Autodesk Fusion 360 part; units mm, degrees
note: some values were not read from the file. Chosen so that the rebuilt part matches the saved one: a direction; which face or edge a step refers to; a side. Set by a fixed rule: which sketch regions a step uses.
(part 2 of 2)
extrude "Extrusion31" cut sketch "Skizze28" against normal blind 1.5 contours L3 A2 A3 | L3 A2 A3 | L3 A3 picked at (-0.3969, 21.4267) bodies 2
sketch "Skizze29" plane through (0, 1.5, 0) normal (0, 1, 0) x (-1, 0, 0)
  line L0 (0.5, -16) -> (0.5, -41)
  line L1 (0.5, -41) -> (35.5, -41)
  line L2 (35.5, -41) -> (35.5, -11)
  line L3 (61, -16) -> (61, -41)
  line L4 (61, -41) -> (67.5, -41)
  line L5 (67.5, -41) -> (67.5, 41)
  line L6 (67.5, 41) -> (38.5, 41)
  line L7 (-67.5, 41) -> (-67.5, -41)
  line L8 (-67.5, -41) -> (-25, -41)
  line L9 (-25, -41) -> (-25, -16)
  line L10 (-25, -16) -> (0.5, -16)
  line L11 (38.5, 33) -> (32.5, 33)
  line L12 (32.5, 33) -> (32.5, 41)
  line L13 (38.5, 41) -> (38.5, 33)
  line L14 (-38.5, -5) -> (-32.5, -5)
  line L15 (-32.5, -5) -> (-32.5, -11)
  line L16 (-38.5, -11) -> (-38.5, -5)
  line L17 (-67.5, -11) -> (-57.5, -11)
  line L18 (-57.5, -11) -> (-57.5, 19)
  line L19 (-57.5, 19) -> (-67.5, 19)
  line L20 (-67.5, 19) -> (-67.5, -11)
  line L21 (-67.5, -11.5) -> (-56.5, -11.5)
  line L22 (-56.5, -11.5) -> (-56.5, -9.5)
  line L23 (-56.5, -9.5) -> (-54.5, -9.5)
  line L24 (-54.5, -9.5) -> (-54.5, -13.5)
  line L25 (-54.5, -13.5) -> (-67.5, -13.5)
  line L26 (-67.5, 19.5) -> (-57, 19.5)
  line L27 (-57, 19.5) -> (-57, 17.5)
  line L28 (-57, 17.5) -> (-55, 17.5)
  line L29 (-55, 17.5) -> (-55, 21.5)
  line L30 (-55, 21.5) -> (-67.5, 21.5)
  line L31 (-38.5, 35) -> (-38.5, 41)
  line L32 (-34.5, 41) -> (-34.5, 35)
  line L33 (-34.5, 35) -> (-38.5, 35)
  line L34 (38.5, -7) -> (38.5, -16)
  line L35 (34.5, -11) -> (34.5, -7)
  line L36 (34.5, -7) -> (38.5, -7)
  line L37 (38.5, -16) -> (61, -16)
  line L38 (32.5, 41) -> (-34.5, 41)
  line L39 (-38.5, 41) -> (-67.5, 41)
  line L40 (35.5, -11) -> (34.5, -11)
  line L41 (-32.5, -11) -> (-38.5, -11)
  dimension "d194" = 1
  dimension "d195" = 0.5
  dimension "d196" = 2
  dimension "d197" = 2
  dimension "d198" = 1.5
  dimension "d199" = 0.5
  dimension "d200" = 0.5
  dimension "d201" = 2
  dimension "d202" = 2
  dimension "d203" = 1.5
  constraint coincident L7 L21.start
  constraint perpendicular L7 L21
  constraint perpendicular L21 L22
  constraint perpendicular L7 L23
  constraint perpendicular L23 L24
  constraint coincident L7 L25.end
  constraint perpendicular L7 L25
  constraint coincident L7 L26.start
  constraint perpendicular L7 L26
  constraint perpendicular L26 L27
  constraint perpendicular L7 L28
  constraint perpendicular L26 L29
  constraint coincident L7 L30.end
  constraint perpendicular L7 L30
  measures "d194" distance of L18 L22
  measures "d195" distance of L17 L21
  measures "d196" distance of L21 L25
  measures "d197" distance of L22 L24
  measures "d198" distance of L17 L23
  measures "d199" distance of L19 L26
  measures "d200" distance of L18 L27
  measures "d201" distance of L26 L30
  measures "d202" distance of L27 L29
  measures "d203" distance of L19 L28
extrude "Extrusion32" add sketch "Skizze29" along normal up to surface (12.5 mm away) contours L7 L21 L22 L23 L24 L25 | L7 L26 L27 L28 L29 L30 bodies 1
sketch "Skizze30" plane through (0, 0, 42.5) normal (0, 0, 1) x (1, 0, 0)
  line L0 (29.5, 41.5) -> (29.5, 34.5)
  line L1 (29.5, 34.5) -> (16.5, 34.5)
  line L2 (16.5, 34.5) -> (16.5, 41.5)
  line L3 (16.5, 41.5) -> (-48, 41.5)
  line L4 (-48, 41.5) -> (-69, 20.5)
  line L5 (-69, 20.5) -> (-69, 14)
  line L6 (-69, 14) -> (69, 14)
  line L7 (69, 14) -> (69, 32.5)
  line L8 (69, 32.5) -> (60, 41.5)
  line L9 (60, 41.5) -> (29.5, 41.5)
  line L10 (-29.7713, 17.8604) -> (-38.3749, 30.1476)
  arc A0 (-38.3749, 30.1476) -> (-40.8324, 28.4269) centre (-39.6036, 29.2873) ccw
  line L11 (-40.8324, 28.4269) -> (-32.2287, 16.1396)
  arc A1 (-32.2287, 16.1396) -> (-29.7713, 17.8604) centre (-31, 17) ccw
  line L12 (-31, 17) -> (-39.6036, 29.2873) construction
  line L13 (-28.8324, 28.4269) -> (-20.2287, 16.1396)
  arc A2 (-26.3749, 30.1476) -> (-28.8324, 28.4269) centre (-27.6036, 29.2873) ccw
  line L14 (-17.7713, 17.8604) -> (-26.3749, 30.1476)
  arc A3 (-20.2287, 16.1396) -> (-17.7713, 17.8604) centre (-19, 17) ccw
  line L15 (-16.8324, 28.4269) -> (-8.2287, 16.1396)
  arc A4 (-14.3749, 30.1476) -> (-16.8324, 28.4269) centre (-15.6036, 29.2873) ccw
  line L16 (-5.7713, 17.8604) -> (-14.3749, 30.1476)
  arc A5 (-8.2287, 16.1396) -> (-5.7713, 17.8604) centre (-7, 17) ccw
  line L17 (-4.8324, 28.4269) -> (3.7713, 16.1396)
  line L18 (6.2287, 17.8604) -> (-2.3749, 30.1476)
  arc A6 (-2.3749, 30.1476) -> (-4.8324, 28.4269) centre (-3.6036, 29.2873) ccw
  arc A7 (3.7713, 16.1396) -> (6.2287, 17.8604) centre (5, 17) ccw
  line L19 (54.2287, 17.8604) -> (45.6251, 30.1476)
  line L20 (43.1676, 28.4269) -> (51.7713, 16.1396)
  arc A8 (51.7713, 16.1396) -> (54.2287, 17.8604) centre (53, 17) ccw
  arc A9 (45.6251, 30.1476) -> (43.1676, 28.4269) centre (44.3964, 29.2873) ccw
  line L21 (42.2287, 17.8604) -> (33.6251, 30.1476)
  line L22 (31.1676, 28.4269) -> (39.7713, 16.1396)
  arc A10 (33.6251, 30.1476) -> (31.1676, 28.4269) centre (32.3964, 29.2873) ccw
  arc A11 (39.7713, 16.1396) -> (42.2287, 17.8604) centre (41, 17) ccw
  line L23 (30.2287, 17.8604) -> (21.6251, 30.1476)
  arc A12 (27.7713, 16.1396) -> (30.2287, 17.8604) centre (29, 17) ccw
  line L24 (19.1676, 28.4269) -> (27.7713, 16.1396)
  arc A13 (21.6251, 30.1476) -> (19.1676, 28.4269) centre (20.3964, 29.2873) ccw
  line L25 (18.2287, 17.8604) -> (9.6251, 30.1476)
  line L26 (7.1676, 28.4269) -> (15.7713, 16.1396)
  arc A14 (15.7713, 16.1396) -> (18.2287, 17.8604) centre (17, 17) ccw
  arc A15 (9.6251, 30.1476) -> (7.1676, 28.4269) centre (8.3964, 29.2873) ccw
  line L27 (-69, 14) -> (69, 14)
  line L28 (69, 14) -> (69, 17)
  line L29 (69, 17) -> (-69, 17)
  line L30 (-69, 17) -> (-69, 14)
  dimension "d206" = 15
  dimension "d207" = 3
  dimension "d208" = 15
  dimension "d209" = 3
  dimension "d210" = 15
  dimension "d211" = 3
  dimension "d212" = 15
  dimension "d213" = 3
  dimension "d214" = 15
  dimension "d215" = 3
  dimension "d216" = 15
  dimension "d217" = 3
  dimension "d218" = 15
  dimension "d219" = 3
  dimension "d220" = 15
  dimension "d221" = 3
  dimension "d222" = 3
  dimension "d224" = 12
  dimension "d225" = 12
  dimension "d226" = 12
  dimension "d227" = 12
  dimension "d228" = 12
  dimension "d229" = 12
  dimension "d230" = 12
  dimension "d231" = 38
  dimension "d234" = 55
  constraint tangent L10 A0
  constraint tangent A0 L11
  constraint parallel L10 L11
  constraint tangent L11 A1
  constraint tangent L10 A1
  constraint tangent A2 L14
  constraint tangent L13 A2
  constraint parallel L13 L14
  constraint tangent L13 A3
  constraint tangent L14 A3
  constraint tangent A4 L16
  constraint tangent L15 A4
  constraint parallel L15 L16
  constraint tangent L15 A5
  constraint tangent L16 A5
  constraint tangent L18 A6
  constraint tangent L17 A6
  constraint parallel L17 L18
  constraint tangent L17 A7
  constraint tangent L18 A7
  constraint tangent L25 A15
  constraint tangent L26 A15
  constraint parallel L25 L26
  constraint tangent L26 A14
  constraint tangent L25 A14
  constraint tangent L23 A13
  constraint tangent L24 A13
  constraint parallel L23 L24
  constraint tangent A12 L24
  constraint tangent L23 A12
  constraint tangent L21 A10
  constraint tangent L22 A10
  constraint parallel L21 L22
  constraint tangent L22 A11
  constraint tangent L21 A11
  constraint tangent L19 A9
  constraint tangent L20 A9
  constraint parallel L19 L20
  constraint tangent L20 A8
  constraint tangent L19 A8
  constraint horizontal L27
  constraint vertical L28
  constraint horizontal L29
  constraint vertical L30
  constraint coincident L7 L28.end
  constraint coincident L5.end L6.start
  constraint coincident A1.centre L29
  constraint coincident A3.centre L29
  constraint coincident A5.centre L29
  constraint coincident A7.centre L29
  constraint coincident A14.centre L29
  constraint coincident A12.centre L29
  constraint coincident A11.centre L29
  constraint coincident A8.centre L29
  constraint parallel L10 L13
  constraint parallel L14 L15
  constraint parallel L16 L17
  constraint parallel L18 L26
  constraint parallel L24 L25
  constraint parallel L22 L23
  constraint parallel L20 L21
  measures "d206" distance of A1.centre A0.centre
  measures "d207" diameter of A0
  measures "d208" distance of A2.centre A3.centre
  measures "d209" diameter of A2
  measures "d210" distance of A4.centre A5.centre
  measures "d211" diameter of A4
  measures "d212" distance of A6.centre A7.centre
  measures "d213" diameter of A6
  measures "d214" distance of A15.centre A14.centre
  measures "d215" diameter of A15
  measures "d216" distance of A13.centre A12.centre
  measures "d217" diameter of A13
  measures "d218" distance of A10.centre A11.centre
  measures "d219" diameter of A10
  measures "d220" distance of A9.centre A8.centre
  measures "d221" diameter of A9
  measures "d222" distance of L27 L29
  measures "d224" distance of A1.centre A3.centre
  measures "d225" distance of A3.centre A5.centre
  measures "d226" distance of A5.centre A7.centre
  measures "d227" distance of A7.centre A14.centre
  measures "d228" distance of A14.centre A12.centre
  measures "d229" distance of A12.centre A11.centre
  measures "d230" distance of A11.centre A8.centre
  measures "d231" distance of A1.centre L29.end
  measures "d234" angle of L11 L29
extrude "Extrusion33" cut sketch "Skizze30" against normal blind 1.5 contours L19 L20 A8 A9 L29 | L20 A8 L29 | L21 L22 A10 A11 L29 | L22 A11 L29 | L11 A1 L29 | L10 A0 L11 A1 L29 | L23 A12 L24 A13 L29 | A12 L24 L29 | L13 A3 L29 | L13 A2 L14 A3 L29 | L25 L26 A14 A15 L29 | L26 A14 L29 | L15 A5 L29 | L15 A4 L16 A5 L29 | L17 L18 A6 A7 L29 | L17 A7 L29 bodies 2
sketch "Skizze34" plane through (0, 0, 42.5) normal (0, 0, 1) x (1, 0, 0)
  line L0 (27.7713, 16.1396) -> (19.1676, 28.4269)
  arc A0 (21.6251, 30.1476) -> (19.1676, 28.4269) centre (20.3964, 29.2873) ccw
  line L1 (21.6251, 30.1476) -> (30.2287, 17.8604)
  arc A1 (27.7713, 16.1396) -> (30.2287, 17.8604) centre (29, 17) ccw
  line L2 (-26.3749, 30.1476) -> (-17.7713, 17.8604)
  arc A2 (-20.2287, 16.1396) -> (-17.7713, 17.8604) centre (-19, 17) ccw
  line L3 (-20.2287, 16.1396) -> (-28.8324, 28.4269)
  arc A3 (-26.3749, 30.1476) -> (-28.8324, 28.4269) centre (-27.6036, 29.2873) ccw
  line L4 (-14.3749, 30.1476) -> (-5.7713, 17.8604)
  arc A4 (-8.2287, 16.1396) -> (-5.7713, 17.8604) centre (-7, 17) ccw
  line L5 (-8.2287, 16.1396) -> (-16.8324, 28.4269)
  arc A5 (-14.3749, 30.1476) -> (-16.8324, 28.4269) centre (-15.6036, 29.2873) ccw
  line L6 (33.6251, 30.1476) -> (42.2287, 17.8604)
  arc A6 (39.7713, 16.1396) -> (42.2287, 17.8604) centre (41, 17) ccw
  line L7 (39.7713, 16.1396) -> (31.1676, 28.4269)
  arc A7 (33.6251, 30.1476) -> (31.1676, 28.4269) centre (32.3964, 29.2873) ccw
  line L8 (15.7713, 16.1396) -> (7.1676, 28.4269)
  arc A8 (9.6251, 30.1476) -> (7.1676, 28.4269) centre (8.3964, 29.2873) ccw
  line L9 (9.6251, 30.1476) -> (18.2287, 17.8604)
  arc A9 (15.7713, 16.1396) -> (18.2287, 17.8604) centre (17, 17) ccw
  line L10 (-38.3749, 30.1476) -> (-29.7713, 17.8604)
  arc A10 (-32.2287, 16.1396) -> (-29.7713, 17.8604) centre (-31, 17) ccw
  line L11 (-32.2287, 16.1396) -> (-40.8324, 28.4269)
  arc A11 (-38.3749, 30.1476) -> (-40.8324, 28.4269) centre (-39.6036, 29.2873) ccw
  line L12 (-2.3749, 30.1476) -> (6.2287, 17.8604)
  arc A12 (3.7713, 16.1396) -> (6.2287, 17.8604) centre (5, 17) ccw
  line L13 (3.7713, 16.1396) -> (-4.8324, 28.4269)
  arc A13 (-2.3749, 30.1476) -> (-4.8324, 28.4269) centre (-3.6036, 29.2873) ccw
  line L14 (51.7713, 16.1396) -> (43.1676, 28.4269)
  arc A14 (45.6251, 30.1476) -> (43.1676, 28.4269) centre (44.3964, 29.2873) ccw
  line L15 (45.6251, 30.1476) -> (54.2287, 17.8604)
  arc A15 (51.7713, 16.1396) -> (54.2287, 17.8604) centre (53, 17) ccw
  line L16 (29.5, 41.5) -> (29.5, 34.5)
  line L17 (29.5, 34.5) -> (16.5, 34.5)
  line L18 (16.5, 34.5) -> (16.5, 41.5)
  line L19 (16.5, 41.5) -> (-48, 41.5)
  line L20 (-48, 41.5) -> (-69, 20.5)
  line L21 (-69, 20.5) -> (-69, 14)
  line L22 (-69, 14) -> (69, 14)
  line L23 (69, 14) -> (69, 32.5)
  line L24 (69, 32.5) -> (60, 41.5)
  line L25 (60, 41.5) -> (29.5, 41.5)
  line L26 (48, 41.5) -> (69, 20.5)
  dimension "d239" = 45
  dimension "d240" = 21
  constraint coincident L25 L26.start
  constraint coincident L23 L26.end
  measures "d239" angle of L25 L26
  measures "d240" distance of L23 L26.start
extrude "Extrusion36" cut sketch "Skizze34" against normal up to surface (22.5 mm away) contours L23 L24 L25 L26 bodies 2
sketch "Skizze35" plane through (0, 0, -42.5) normal (0, 0, -1) x (-1, 0, 0)
  line L0 (11.7592, 31.0652) -> (2.0084, 17.1396)
  arc A0 (-0.449, 18.8604) -> (2.0084, 17.1396) centre (0.7797, 18) ccw
  line L1 (-0.449, 18.8604) -> (9.3018, 32.7859)
  arc A1 (11.7592, 31.0652) -> (9.3018, 32.7859) centre (10.5305, 31.9256) ccw
  line L2 (-24.4169, 31.0652) -> (-34.1677, 17.1396)
  arc A2 (-36.6251, 18.8604) -> (-34.1677, 17.1396) centre (-35.3964, 18) ccw
  line L3 (-36.6251, 18.8604) -> (-26.8743, 32.7859)
  arc A3 (-24.4169, 31.0652) -> (-26.8743, 32.7859) centre (-25.6456, 31.9256) ccw
  arc A4 (23.4355, 31.0652) -> (20.978, 32.7859) centre (22.2067, 31.9256) ccw
  line L4 (23.4355, 31.0652) -> (13.6847, 17.1396)
  arc A5 (11.2272, 18.8604) -> (13.6847, 17.1396) centre (12.4559, 18) ccw
  line L5 (11.2272, 18.8604) -> (20.978, 32.7859)
  line L6 (-12.4933, 18.8604) -> (-2.7425, 32.7859)
  arc A6 (-0.285, 31.0652) -> (-2.7425, 32.7859) centre (-1.5137, 31.9256) ccw
  line L7 (-0.285, 31.0652) -> (-10.0358, 17.1396)
  arc A7 (-12.4933, 18.8604) -> (-10.0358, 17.1396) centre (-11.2645, 18) ccw
  line L8 (-12.202, 31.0652) -> (-21.9528, 17.1396)
  arc A8 (-24.4103, 18.8604) -> (-21.9528, 17.1396) centre (-23.1816, 18) ccw
  line L9 (-24.4103, 18.8604) -> (-14.6595, 32.7859)
  arc A9 (-12.202, 31.0652) -> (-14.6595, 32.7859) centre (-13.4308, 31.9256) ccw
  arc A10 (35.8961, 31.0652) -> (33.4386, 32.7859) centre (34.6674, 31.9256) ccw
  line L10 (35.8961, 31.0652) -> (26.1453, 17.1396)
  arc A11 (23.6878, 18.8604) -> (26.1453, 17.1396) centre (24.9166, 18) ccw
  line L11 (23.6878, 18.8604) -> (33.4386, 32.7859)
  line L12 (-69, 32.5) -> (-69, 14)
  line L13 (-69, 14) -> (69, 14)
  line L14 (69, 14) -> (69, 20.5)
  line L15 (69, 20.5) -> (48, 41.5)
  line L16 (48, 41.5) -> (-60, 41.5)
  line L17 (-60, 41.5) -> (-69, 32.5)
  line L18 (-48, 41.5) -> (-69, 20.5)
  dimension "d243" = 45
  dimension "d244" = 21
  constraint coincident L16 L18.start
  constraint coincident L12 L18.end
  measures "d243" angle of L16 L18
  measures "d244" distance of L12 L18.start
extrude "Extrusion37" cut sketch "Skizze35" against normal up to surface (30.5 mm away) contours L12 L16 L17 L18 bodies 2
sketch "Skizze36" plane through (44.75, 44.75, 0) normal (0.707107, 0.707107, 0) x (0, 0, -1)
  line L0 (-41, -6.7175) -> (-20, -6.7175)
  line L1 (-20, -6.7175) -> (-20, -4.5962)
  line L2 (-20, -4.5962) -> (-42.5, -4.5962)
  line L3 (-42.5, -4.5962) -> (-42.5, -34.2947)
  line L4 (-42.5, -34.2947) -> (-20, -34.2947)
  line L5 (-20, -34.2947) -> (-20, -32.1734)
  line L6 (-20, -32.1734) -> (-41, -32.1734)
  line L7 (-41, -32.1734) -> (-41, -6.7175)
  line L8 (-42.5, -4.5962) -> (-20, -4.5962)
  line L9 (-20, -4.5962) -> (-20, -34.2947)
  line L10 (-20, -34.2947) -> (-42.5, -34.2947)
  line L11 (-42.5, -34.2947) -> (-42.5, -4.5962)
  line L12 (12, -6.7175) -> (41, -6.7175)
  line L13 (41, -6.7175) -> (41, -32.1734)
  line L14 (41, -32.1734) -> (12, -32.1734)
  line L15 (12, -32.1734) -> (12, -34.2947)
  line L16 (12, -34.2947) -> (42.5, -34.2947)
  line L17 (42.5, -34.2947) -> (42.5, -4.5962)
  line L18 (42.5, -4.5962) -> (12, -4.5962)
  line L19 (12, -4.5962) -> (12, -6.7175)
  line L20 (12, -4.5962) -> (42.5, -4.5962)
  line L21 (42.5, -4.5962) -> (42.5, -34.2947)
  line L22 (42.5, -34.2947) -> (12, -34.2947)
  line L23 (12, -34.2947) -> (12, -4.5962)
  constraint horizontal L8
  constraint vertical L9
  constraint horizontal L10
  constraint vertical L11
  constraint coincident L4.end L5.start
  constraint coincident L2.end L3.start
  constraint horizontal L20
  constraint vertical L21
  constraint horizontal L22
  constraint vertical L23
  constraint coincident L16.end L17.start
  constraint coincident L18.end L19.start
extrude "Extrusion38" add sketch "Skizze36" against normal blind 1.5 bodies 2
sketch "Skizze37" plane through (0, 0, 20) normal (0, 0, 1) x (1, 0, 0)
  line L0 (49.5, 40) -> (59.3787, 40)
  line L1 (59.3787, 40) -> (67.5, 31.8787)
  line L2 (67.5, 31.8787) -> (67.5, 22)
  line L3 (67.5, 22) -> (69, 20.5)
  line L4 (69, 20.5) -> (69, 32.5)
  line L5 (69, 32.5) -> (60, 41.5)
  line L6 (60, 41.5) -> (48, 41.5)
  line L7 (48, 41.5) -> (49.5, 40)
  line L8 (49.5, 40) -> (67.5, 22)
extrude "Extrusion39" add sketch "Skizze37" along normal blind 1.5 bodies 2
sketch "Skizze38" plane through (0, 0, -12) normal (0, 0, -1) x (-1, 0, 0)
  line L0 (-59.3787, 40) -> (-49.5, 40)
  line L1 (-49.5, 40) -> (-48, 41.5)
  line L2 (-48, 41.5) -> (-60, 41.5)
  line L3 (-60, 41.5) -> (-69, 32.5)
  line L4 (-69, 32.5) -> (-69, 20.5)
  line L5 (-69, 20.5) -> (-67.5, 22)
  line L6 (-67.5, 22) -> (-67.5, 31.8787)
  line L7 (-67.5, 31.8787) -> (-59.3787, 40)
  line L8 (-67.5, 22) -> (-49.5, 40)
extrude "Extrusion40" add sketch "Skizze38" along normal blind 1.5 bodies 2
sketch "Skizze39" plane through (0, 1.5, 0) normal (0, 1, 0) x (-1, 0, 0)
  line L0 (-57, 19.5) -> (-67.5, 19.5)
  line L1 (-67.5, 19.5) -> (-67.5, -11.5)
  line L2 (-67.5, -11.5) -> (-56.5, -11.5)
  line L3 (-56.5, -11.5) -> (-56.5, -9.5)
  line L4 (-56.5, -9.5) -> (-54.5, -9.5)
  line L5 (-54.5, -9.5) -> (-54.5, -13.5)
  line L6 (-54.5, -13.5) -> (-67.5, -13.5)
  line L7 (-67.5, -13.5) -> (-67.5, -41)
  line L8 (-67.5, -41) -> (-25, -41)
  line L9 (-25, -41) -> (-25, -16)
  line L10 (-25, -16) -> (0.5, -16)
  line L11 (0.5, -16) -> (0.5, -41)
  line L12 (0.5, -41) -> (35.5, -41)
  line L13 (35.5, -41) -> (35.5, -11)
  line L14 (61, -16) -> (61, -41)
  line L15 (61, -41) -> (67.5, -41)
  line L16 (67.5, -41) -> (67.5, 41)
  line L17 (67.5, 41) -> (38.5, 41)
  line L18 (-67.5, 41) -> (-67.5, 21.5)
  line L19 (-67.5, 21.5) -> (-55, 21.5)
  line L20 (-55, 21.5) -> (-55, 17.5)
  line L21 (-55, 17.5) -> (-57, 17.5)
  line L22 (-57, 17.5) -> (-57, 19.5)
  line L23 (-38.5, -5) -> (-32.5, -5)
  line L24 (-32.5, -5) -> (-32.5, -11)
  line L25 (-38.5, -11) -> (-38.5, -5)
  line L26 (38.5, 33) -> (32.5, 33)
  line L27 (32.5, 33) -> (32.5, 41)
  line L28 (38.5, 41) -> (38.5, 33)
  line L29 (67.5, 41) -> (61.5, 41)
  line L30 (61.5, 41) -> (61.5, 36)
  line L31 (61.5, 36) -> (67.5, 36)
  line L32 (67.5, 36) -> (67.5, 41)
  circle A0 centre (64.5, 38.5) radius 1.6
  line L33 (0, 1.75) -> (0, 22.5)
  line L34 (-61.5, 41) -> (-61.5, 36)
  line L35 (-61.5, 36) -> (-67.5, 36)
  circle A1 centre (-64.5, 38.5) radius 1.6
  line L36 (-67.5, 41) -> (-61.5, 41)
  line L37 (-67.5, 36) -> (-67.5, 41)
  line L38 (-1.75, 0) -> (-22.5, 0)
  line L39 (61.5, -36) -> (67.5, -36)
  circle A2 centre (64.5, -38.5) radius 1.6
  line L40 (61.5, -41) -> (61.5, -36)
  line L41 (67.5, -41) -> (61.5, -41)
  line L42 (67.5, -36) -> (67.5, -41)
  line L43 (-61.5, -41) -> (-61.5, -36)
  line L44 (-61.5, -36) -> (-67.5, -36)
  line L45 (-67.5, -36) -> (-67.5, -41)
  line L46 (-67.5, -41) -> (-61.5, -41)
  circle A3 centre (-64.5, -38.5) radius 1.6
  line L47 (38.5, -7) -> (38.5, -16)
  line L48 (34.5, -11) -> (34.5, -7)
  line L49 (34.5, -7) -> (38.5, -7)
  line L50 (-38.5, 35) -> (-38.5, 41)
  line L51 (-34.5, 41) -> (-34.5, 35)
  line L52 (-34.5, 35) -> (-38.5, 35)
  line L53 (38.5, -16) -> (61, -16)
  line L54 (32.5, 41) -> (-34.5, 41)
  line L55 (-38.5, 41) -> (-67.5, 41)
  line L56 (35.5, -11) -> (34.5, -11)
  line L57 (-32.5, -11) -> (-38.5, -11)
  point P0 (-64.5, -38.5)
  point P1 (-64.5, -38.5)
  dimension "d253" = 6
  dimension "d254" = 5
  dimension "d255" = 3.2
  dimension "d256" = 3
  dimension "d257" = 2.5
  constraint horizontal L29
  constraint vertical L30
  constraint horizontal L31
  constraint vertical L32
  constraint coincident L16.end L17.start
  constraint symmetric L16.end L33 L18.start
  constraint symmetric L29.end L33 L34.start
  constraint symmetric L30.end L33 L34.end
  constraint symmetric L31.end L33 L35.end
  constraint symmetric A0 L33 A1
  constraint symmetric L16.end L38 L15.end
  constraint symmetric L29.end L38 L40.start
  constraint symmetric L30.end L38 L39.start
  constraint symmetric L31.end L38 L39.end
  constraint symmetric A0 L38 A2
  constraint symmetric L34.start L38 L43.start
  constraint symmetric L34.end L38 L43.end
  constraint symmetric L35.end L38 L44.end
  constraint symmetric A1.centre L38 P1
  constraint symmetric L18.start L38 L7.end
  constraint symmetric A1 L38 A3
  measures "d253" distance of L30.end L31.end
  measures "d254" distance of L29.end L30.end
  measures "d255" diameter of A0
  measures "d256" distance of L32 A0.centre
  measures "d257" distance of L31 A0.centre
extrude "Extrusion41" add sketch "Skizze39" along normal up to surface (11 mm away) contours L18 L34 L35 L36 L37 L55 | L7 L8 L43 L44 L45 L46 | L16 L17 L29 L30 L31 L32 | L15 L16 L39 L40 L41 L42 bodies 1
extrude "Extrusion58" cut 4 faces at (64.7139, 1.5, 38.603) (64.7139, 1.5, -38.397) (-64.1384, 1.5, 39.3056) (-64.1384, 1.5, -37.6944) along direction (0, 1, 0) up to surface end surface through (0, 0, 0) normal (0, -1, 0) offset 0 on bodies 1 bodies 1
sketch "Skizze54" plane through (0, 1.5, 0) normal (0, 1, 0) x (-1, 0, 0)
  line L0 (-61.5, 36) -> (-67.5, 36)
  line L1 (-67.5, 36) -> (-67.5, 21.5)
  line L2 (-67.5, 21.5) -> (-55, 21.5)
  line L3 (-55, 21.5) -> (-55, 17.5)
  line L4 (-55, 17.5) -> (-57, 17.5)
  line L5 (-57, 17.5) -> (-57, 19.5)
  line L6 (-57, 19.5) -> (-67.5, 19.5)
  line L7 (-67.5, 19.5) -> (-67.5, -11.5)
  line L8 (-67.5, -11.5) -> (-56.5, -11.5)
  line L9 (-56.5, -11.5) -> (-56.5, -9.5)
  line L10 (-56.5, -9.5) -> (-54.5, -9.5)
  line L11 (-54.5, -9.5) -> (-54.5, -13.5)
  line L12 (-54.5, -13.5) -> (-67.5, -13.5)
  line L13 (-67.5, -13.5) -> (-67.5, -36)
  line L14 (-67.5, -36) -> (-61.5, -36)
  line L15 (-61.5, -36) -> (-61.5, -41)
  line L16 (-61.5, -41) -> (-25, -41)
  line L17 (-25, -41) -> (-25, -16)
  line L18 (-25, -16) -> (0.5, -16)
  line L19 (0.5, -16) -> (0.5, -41)
  line L20 (0.5, -41) -> (35.5, -41)
  line L21 (35.5, -41) -> (35.5, -11)
  line L22 (61, -16) -> (61, -41)
  line L23 (61, -41) -> (61.5, -41)
  line L24 (61.5, -41) -> (61.5, -36)
  line L25 (61.5, -36) -> (67.5, -36)
  line L26 (67.5, -36) -> (67.5, 36)
  line L27 (67.5, 36) -> (61.5, 36)
  line L28 (61.5, 36) -> (61.5, 41)
  line L29 (61.5, 41) -> (38.5, 41)
  line L30 (-61.5, 41) -> (-61.5, 36)
  line L31 (-38.5, 35) -> (-38.5, 41)
  line L32 (-34.5, 41) -> (-34.5, 35)
  line L33 (-34.5, 35) -> (-38.5, 35)
  line L34 (38.5, -7) -> (38.5, -16)
  line L35 (34.5, -11) -> (34.5, -7)
  line L36 (34.5, -7) -> (38.5, -7)
  line L37 (38.5, 33) -> (32.5, 33)
  line L38 (32.5, 33) -> (32.5, 41)
  line L39 (38.5, 41) -> (38.5, 33)
  line L40 (-38.5, -5) -> (-32.5, -5)
  line L41 (-32.5, -5) -> (-32.5, -11)
  line L42 (-38.5, -11) -> (-38.5, -5)
  line L43 (67.5, -34) -> (59.5, -34)
  line L44 (59.5, -34) -> (59.5, -41)
  line L45 (67.5, 34) -> (59.5, 34)
  line L46 (59.5, 34) -> (59.5, 41)
  line L47 (-59.5, 41) -> (-59.5, 34)
  line L48 (-59.5, 34) -> (-67.5, 34)
  line L49 (-67.5, -34) -> (-59.5, -34)
  line L50 (-59.5, -34) -> (-59.5, -41)
  line L51 (38.5, -16) -> (61, -16)
  line L52 (32.5, 41) -> (-34.5, 41)
  line L53 (-38.5, 41) -> (-61.5, 41)
  line L54 (35.5, -11) -> (34.5, -11)
  line L55 (-32.5, -11) -> (-38.5, -11)
  dimension "d340" = 2
  dimension "d341" = 2
  dimension "d342" = 2
  dimension "d343" = 2
  dimension "d344" = 2
  dimension "d345" = 2
  dimension "d346" = 2
  dimension "d347" = 2
  constraint coincident L26 L43.start
  constraint perpendicular L26 L43
  constraint coincident L23 L44.end
  constraint perpendicular L23 L44
  constraint coincident L26 L45.start
  constraint perpendicular L26 L45
  constraint coincident L29 L46.end
  constraint perpendicular L29 L46
  constraint coincident L29 L47.start
  constraint perpendicular L29 L47
  constraint coincident L1 L48.end
  constraint perpendicular L1 L48
  constraint coincident L13 L49.start
  constraint perpendicular L13 L49
  constraint coincident L16 L50.end
  constraint perpendicular L16 L50
  measures "d340" distance of L24 L44
  measures "d341" distance of L25 L43
  measures "d342" distance of L28 L46
  measures "d343" distance of L27 L45
  measures "d344" distance of L0 L48
  measures "d345" distance of L30 L47
  measures "d346" distance of L15 L50
  measures "d347" distance of L14 L49
extrude "Extrusion66" add sketch "Skizze54" along normal blind 3 contours L0 L1 L30 L47 L48 L53 | L26 L27 L28 L29 L45 L46 | L22 L23 L24 L25 L26 L43 | L13 L14 L15 L16 L49 L50 bodies 1
sketch "Skizze53" plane through (0, 0, 0) normal (0, -1, 0) x (1, 0, 0)
  circle A0 centre (-64.5, 38.5) radius 1.6
  circle A1 centre (64.5, 38.5) radius 1.6
  circle A2 centre (64.5, -38.5) radius 1.6
  circle A3 centre (-64.5, -38.5) radius 1.6
  line L0 (-69, 42.5) -> (-69, -42.5)
  line L1 (-69, -42.5) -> (69, -42.5)
  line L2 (69, -42.5) -> (69, 42.5)
  line L3 (69, 42.5) -> (-69, 42.5)
  circle A4 centre (-64.5, 38.5) radius 3.1
  circle A5 centre (64.5, 38.5) radius 3.1
  circle A6 centre (-64.5, -38.5) radius 3.1
  circle A7 centre (64.5, -38.5) radius 3.1
  dimension "d337" = 6.2
  constraint concentric A0 A4
  constraint concentric A1 A5
  constraint equal A4 A5
  constraint concentric A3 A6
  constraint concentric A2 A7
  constraint equal A4 A6
  constraint equal A4 A7
  measures "d337" diameter of A4
extrude "Extrusion65" cut sketch "Skizze53" against normal blind 2.1 contours A4 | A5 | A6 | A7 bodies 1
chamfer "Fase7" distance 1.5 angle 45 4 edges at (-63.0083, 2.1, 39.0786) (-63.0083, 2.1, -37.9214) (65.9917, 2.1, -37.9214) (65.9917, 2.1, 39.0786) on bodies 1
sketch "Skizze40" plane through (0, 14, 0) normal (0, -1, 0) x (1, 0, 0)
  line L0 (67.5, 35.25) -> (69, 35.25)
  line L1 (69, 35.25) -> (69, 42.5)
  line L2 (69, 42.5) -> (-69, 42.5)
  line L3 (-69, 42.5) -> (-69, 2)
  line L4 (-69, 2) -> (-67.5, 2)
  line L5 (-67.5, 2) -> (-67.5, 41)
  line L6 (-67.5, 41) -> (67.5, 41)
  line L7 (67.5, 41) -> (67.5, 35.25)
  circle A0 centre (-64.5, -38.5) radius 1.6
  line L8 (-67.5, -36) -> (-61.5, -36)
  line L9 (-61.5, -36) -> (-61.5, -41)
  circle A1 centre (-64.5, 38.5) radius 1.6
  line L10 (-61.5, 41) -> (-61.5, 36)
  line L11 (-61.5, 36) -> (-67.5, 36)
  line L12 (67.5, 36) -> (61.5, 36)
  circle A2 centre (64.5, 38.5) radius 1.6
  line L13 (67.5, 36) -> (61.5, 36)
  line L14 (61.5, 36) -> (61.5, 41)
  circle A3 centre (64.5, -38.5) radius 1.6
  line L15 (61.5, -41) -> (61.5, -36)
  line L16 (61.5, -36) -> (67.5, -36)
  circle A4 centre (-64.5, -38.5) radius 1.35
  line L17 (1.75, 0) -> (22.5, 0)
  circle A5 centre (-64.5, 38.5) radius 1.35
  line L18 (0, 1.75) -> (0, 22.5)
  circle A6 centre (64.5, -38.5) radius 1.35
  circle A7 centre (64.5, 38.5) radius 1.35
  line L19 (-67.5, -41) -> (-67.5, -36)
  line L20 (-61.5, -41) -> (-67.5, -41)
  line L21 (-67.5, 36) -> (-67.5, 41)
  line L22 (-67.5, 41) -> (-61.5, 41)
  line L23 (67.5, 41) -> (67.5, 36)
  line L24 (61.5, 41) -> (67.5, 41)
  line L25 (67.5, -36) -> (67.5, -41)
  line L26 (67.5, -41) -> (61.5, -41)
  dimension "d260" = 2.7
  constraint concentric A0 A4
  constraint symmetric A4 L17 A5
  constraint symmetric A4 L18 A6
  constraint symmetric A5 L18 A7
  measures "d260" diameter of A4
extrude "Extrusion42" add sketch "Skizze40" against normal blind 14 contours L6 L7 L12 L13 L14 L23 L24 | L5 L6 L10 L11 L21 L22 | A0 | L8 L9 L19 L20 | A1 | A2 | A3 | L15 L16 L25 L26 | A4 | A5 | A6 | A7 bodies 2
extrude "Extrusion63" cut sketch "Skizze40" against normal blind 8 contours A4 | A5 | A6 | A7 bodies 2
extrude "Extrusion59" cut 1 faces at (-65.5, 26, 41) along direction (0, 0, -1) up to surface (82 mm away) on bodies 2 bodies 2
extrude "Extrusion60" cut 1 faces at (65.5, 26, -41) along direction (0, 0, 1) blind 5 on bodies 2 bodies 2
extrude "Extrusion61" cut 1 faces at (65.5, 26, 41) along direction (0, 0, -1) up to surface (5 mm away) on bodies 2 bodies 2
sketch "Skizze52" plane through (0, 14, 0) normal (0, -1, 0) x (1, 0, 0)
  circle A0 centre (-64.5, -38.5) radius 1.35
  circle A1 centre (64.5, -38.5) radius 1.35
  line L0 (69, -32) -> (67.5, -32)
  line L1 (67.5, -32) -> (67.5, -36)
  line L2 (67.5, -36) -> (61.5, -36)
  line L3 (61.5, -36) -> (61.5, -41)
  line L4 (61.5, -41) -> (-9.5, -41)
  line L5 (-61.5, -41) -> (-61.5, -36)
  line L6 (-61.5, -36) -> (-67.5, -36)
  line L7 (-67.5, -36) -> (-67.5, -32)
  line L8 (-67.5, -32) -> (-69, -32)
  line L9 (-69, -32) -> (-69, -42.5)
  line L10 (-69, -42.5) -> (69, -42.5)
  line L11 (69, -42.5) -> (69, -32)
  circle A2 centre (-64.5, 38.5) radius 1.35
  circle A3 centre (64.5, 38.5) radius 1.35
  line L12 (67.5, 35.25) -> (69, 35.25)
  line L13 (69, 35.25) -> (69, 42.5)
  line L14 (69, 42.5) -> (-69, 42.5)
  line L15 (-69, 42.5) -> (-69, 2)
  line L16 (-69, 2) -> (-67.5, 2)
  line L17 (-67.5, 2) -> (-67.5, 36)
  line L18 (-67.5, 36) -> (-61.5, 36)
  line L19 (-61.5, 36) -> (-61.5, 41)
  line L20 (-61.5, 41) -> (61.5, 41)
  line L21 (61.5, 41) -> (61.5, 36)
  line L22 (61.5, 36) -> (67.5, 36)
  line L23 (67.5, 36) -> (67.5, 35.25)
  line L24 (-61.5, -36) -> (-67, -36)
  line L25 (-67, -36) -> (-67, -40.5)
  line L26 (-67, -40.5) -> (-61.5, -40.5)
  line L27 (-61.5, -40.5) -> (-61.5, -36)
  line L28 (61.5, -40.5) -> (67, -40.5)
  line L29 (67, -40.5) -> (67, -36)
  line L30 (-61.5, 40.5) -> (-67, 40.5)
  line L31 (-67, 40.5) -> (-67, 36)
  line L32 (61.5, 40.5) -> (67, 40.5)
  line L33 (67, 40.5) -> (67, 36)
  line L34 (-9.5, -41) -> (-9.5, -21)
  line L35 (-9.5, -21) -> (-24.5, -21)
  line L36 (-24.5, -21) -> (-24.5, -41)
  line L37 (-24.5, -41) -> (-61.5, -41)
  dimension "d325" = 0.5
  dimension "d326" = 0.5
  dimension "d328" = 0.5
  dimension "d330" = 0.5
  dimension "d331" = 0.5
  dimension "d332" = 0.5
  dimension "d333" = 0.5
  constraint horizontal L24
  constraint vertical L25
  constraint horizontal L26
  constraint vertical L27
  constraint coincident L5.end L6.start
  constraint coincident L3 L28.start
  constraint perpendicular L3 L28
  constraint coincident L2 L29.end
  constraint perpendicular L2 L29
  constraint coincident L19 L30.start
  constraint perpendicular L19 L30
  constraint coincident L18 L31.end
  constraint perpendicular L18 L31
  constraint coincident L21 L32.start
  constraint perpendicular L21 L32
  constraint coincident L22 L33.end
  constraint perpendicular L22 L33
  measures "d325" distance of L7 L25
  measures "d326" distance of L4 L26
  measures "d328" distance of L1 L29
  measures "d330" distance of L20 L30
  measures "d331" distance of L17 L31
  measures "d332" distance of L20 L32
  measures "d333" distance of L23 L33
extrude "Extrusion64" add sketch "Skizze52" along normal blind 1 contours L2 L3 L28 L29 | L5 L6 L24 L25 L26 L27 | L21 L22 L32 L33 | L18 L19 L30 L31 bodies 2
chamfer "Fase6" distance 1.4 angle 40 4 edges at (-13.1, 41.5, -4.5) (-27, 41.5, 4) (-13.1, 41.5, 12.5) (0.8, 41.5, 4) measured on face at (-26.3129, 41.5, 28.4399) measured on face at (-26.3129, 41.5, 28.4399) measured on face at (-26.3129, 41.5, 28.4399) measured on face at (-26.3129, 41.5, 28.4399) on bodies 2
sketch "Skizze56" plane through (0, 41.5, 0) normal (0, 1, 0) x (-1, 0, 0)
  circle A0 centre (-1.5, 29.5) radius 5.5
  line L0 (38.5, 3.2) -> (38.5, -4.8)
  line L1 (38.5, -4.8) -> (32, -4.8)
  line L2 (32, -4.8) -> (32, 3.2)
  line L3 (32, 3.2) -> (38.5, 3.2)
  line L4 (-27, -2) -> (-19, -2)
  line L5 (-19, -2) -> (-19, -8)
  line L6 (-19, -8) -> (-27, -8)
  line L7 (-27, -8) -> (-27, -2)
  line L8 (-33, -36.5) -> (-33, -16.5)
  line L9 (-33, -16.5) -> (-30, -16.5)
  line L10 (-30, -16.5) -> (-30, -36.5)
  line L11 (-30, -36.5) -> (-33, -36.5)
  line L12 (3, -16.5) -> (6, -16.5)
  line L13 (6, -16.5) -> (6, -36.5)
  line L14 (6, -36.5) -> (3, -36.5)
  line L15 (3, -36.5) -> (3, -16.5)
  line L16 (30, -16.5) -> (33, -16.5)
  line L17 (33, -16.5) -> (33, -36.5)
  line L18 (33, -36.5) -> (30, -36.5)
  line L19 (30, -36.5) -> (30, -16.5)
  line L20 (-3, -16.5) -> (-3, -36.5)
  line L21 (-3, -36.5) -> (-6, -36.5)
  line L22 (-6, -36.5) -> (-6, -16.5)
  line L23 (-6, -16.5) -> (-3, -16.5)
  line L24 (-24, -36.5) -> (-24, -16.5)
  line L25 (-24, -16.5) -> (-21, -16.5)
  line L26 (-21, -16.5) -> (-21, -36.5)
  line L27 (-21, -36.5) -> (-24, -36.5)
  line L28 (12, -16.5) -> (15, -16.5)
  line L29 (15, -16.5) -> (15, -36.5)
  line L30 (15, -36.5) -> (12, -36.5)
  line L31 (12, -36.5) -> (12, -16.5)
  line L32 (21, -16.5) -> (24, -16.5)
  line L33 (24, -16.5) -> (24, -36.5)
  line L34 (24, -36.5) -> (21, -36.5)
  line L35 (21, -36.5) -> (21, -16.5)
  line L36 (-15, -16.5) -> (-12, -16.5)
  line L37 (-12, -16.5) -> (-12, -36.5)
  line L38 (-12, -36.5) -> (-15, -36.5)
  line L39 (-15, -36.5) -> (-15, -16.5)
  line L40 (-48, -13.5) -> (-48, -42.5)
  line L41 (-48, -42.5) -> (48, -42.5)
  line L42 (48, -42.5) -> (48, 42.5)
  line L43 (48, 42.5) -> (-16.5, 42.5)
  line L44 (-16.5, 42.5) -> (-16.5, 36.5)
  line L45 (-16.5, 36.5) -> (-18.5, 36.5)
  line L46 (-18.5, 36.5) -> (-18.5, 27.5)
  line L47 (-18.5, 27.5) -> (-27.5, 27.5)
  line L48 (-27.5, 27.5) -> (-27.5, 36.5)
  line L49 (-27.5, 36.5) -> (-29.5, 36.5)
  line L50 (-29.5, 36.5) -> (-29.5, 42.5)
  line L51 (-29.5, 42.5) -> (-48, 42.5)
  line L52 (-48, 42.5) -> (-48, 21.5)
  line L53 (-48, 21.5) -> (-60, 21.5)
  line L54 (-60, 21.5) -> (-60, -13.5)
  line L55 (-60, -13.5) -> (-48, -13.5)
  line L56 (-2.2, -5.9) -> (-2.2, 13.9)
  line L57 (-2.2, 13.9) -> (28.4, 13.9)
  line L58 (28.4, 13.9) -> (28.4, -5.9)
  line L59 (28.4, -5.9) -> (-2.2, -5.9)
  line L60 (-69, 18.2829) -> (-67.5, 18.2829)
  line L61 (-67.5, 18.2829) -> (-67.5, 19.5)
  line L62 (-67.5, 19.5) -> (-57, 19.5)
  line L63 (-57, 19.5) -> (-57, 17.5)
  line L64 (-57, 17.5) -> (-55, 17.5)
  line L65 (-55, 17.5) -> (-55, 21.5)
  line L66 (-55, 21.5) -> (-67.5, 21.5)
  line L67 (-67.5, 21.5) -> (-67.5, 26.75)
  line L68 (-67.5, 26.75) -> (-69, 26.75)
  line L69 (-69, 26.75) -> (-69, 18.2829)
  line L70 (-67.5, -10.2829) -> (-69, -10.2829)
  line L71 (-69, -10.2829) -> (-69, -23)
  line L72 (-69, -23) -> (-67.5, -23)
  line L73 (-67.5, -23) -> (-67.5, -13.5)
  line L74 (-67.5, -13.5) -> (-54.5, -13.5)
  line L75 (-54.5, -13.5) -> (-54.5, -9.5)
  line L76 (-54.5, -9.5) -> (-56.5, -9.5)
  line L77 (-56.5, -9.5) -> (-56.5, -11.5)
  line L78 (-56.5, -11.5) -> (-67.5, -11.5)
  line L79 (-67.5, -11.5) -> (-67.5, -10.2829)
  line L80 (-67.5, 21.5) -> (-67.5, 19.5)
  line L81 (-67.5, -11.5) -> (-67.5, -13.5)
  line L82 (-26.5, 11.5) -> (-19.5, 11.5)
  line L83 (-19.5, 11.5) -> (-19.5, 7.5)
  line L84 (-19.5, 7.5) -> (-26.5, 7.5)
  line L85 (-26.5, 7.5) -> (-26.5, 11.5)
  constraint coincident L66.end L67.start
  constraint coincident L61.end L62.start
  constraint coincident L78.end L79.start
  constraint coincident L73.end L74.start
extrude "Extrusion67" add sketch "Skizze56" against normal up to surface (26.5 mm away) contours L54 L55 L74 L75 L76 L77 L78 | L54 L74 L78 L81 | L54 L62 L66 L80 | L53 L54 L62 L63 L64 L65 L66 bodies 2
extrude "Extrusion68" cut 1 faces at (65, 39, 19.5) along direction (0, 0, -1) up to surface (33 mm away) and the other way up to surface (2 mm away) on bodies 2 bodies 2
sketch "Skizze59" plane through (69, 0, 0) normal (1, 0, 0) x (0, 0, -1)
  arc A0 (-18.2829, 14) -> (10.2829, 14) centre (-4, 16.5) ccw
  line L0 (-18.2829, 14) -> (-26.75, 14)
  arc A1 (-35.25, 14) -> (-26.75, 14) centre (-31, 14) ccw
  line L1 (-35.25, 14) -> (-42.5, 14)
  line L2 (-42.5, 14) -> (-42.5, 0)
  line L3 (-42.5, 0) -> (42.5, 0)
  line L4 (42.5, 0) -> (42.5, 14)
  line L5 (42.5, 14) -> (32, 14)
  arc A2 (23, 14) -> (32, 14) centre (27.5, 14) ccw
  line L6 (23, 14) -> (10.2829, 14)
  line L7 (-31, 14) -> (-31, 3.3255) construction
  circle A3 centre (-31, 12.5) radius 4.25
  line L8 (-41, 14) -> (-2, 14)
  line L9 (-35.25, 14) -> (-35.25, 12.5)
  line L10 (-26.75, 14) -> (-26.75, 12.5)
  dimension "d378" = 8.5
  dimension "d379" = 1.5
  constraint coincident A1.centre L7.start
  constraint vertical L7
  constraint coincident L7 A3.centre
  constraint coincident A1.start L1.start
  constraint coincident A3 L9.end
  constraint tangent A3 L9
  constraint coincident L0.end A1.end
  constraint coincident A3 L10.end
  constraint tangent A3 L10
  measures "d378" diameter of A3
  measures "d379" distance of A3.centre L8
extrude "Extrusion74" cut sketch "Skizze59" against normal blind 1.5 contours A1 A3 L10 | A1 A3 | A1 A3 L9 bodies 1
extrude "Extrusion80" cut 1 faces at (-35.5, 3.1667, -21) along direction (-1, 0, 0) blind 2 on bodies 1 bodies 1
extrude "Extrusion81" cut 1 faces at (-0.5, 4.8333, -32.6667) along direction (1, 0, 0) blind 2 on bodies 1 bodies 1
extrude "Extrusion82" cut 1 faces at (24.1667, 41, 7.5) along direction (0, 0, -1) blind 2 on bodies 2 bodies 2
equation "d9 = d8"
equation "d11 = d10"
equation "d12 = d10"
equation "d13 = d10"
equation "d39 = d38"
equation "d40 = d38"
equation "d41 = d38"
equation "d81 = d80"
equation "d82 = d80"
equation "d83 = d80"
equation "d128 = d126"
equation "d129 = d127"
equation "d130 = d127"
equation "d131 = d126"
equation "d132 = d127"
equation "d133 = d126"
equation "d137 = d136"
equation "d138 = d136"
equation "d148 = d146"
equation "d150 = d146"
equation "d155 = d145"
equation "d156 = d145"
equation "d170 = d169"
equation "d171 = d169"
equation "d172 = d169"
equation "d199 = d195"
equation "d200 = d195"
equation "d201 = d196"
equation "d202 = d197"
equation "d203 = d198"
equation "d225 = d224"
equation "d226 = d224"
equation "d227 = d224"
equation "d228 = d224"
equation "d229 = d224"
equation "d230 = d224"
equation "d256 = d253 / 2"
equation "d257 = d254 / 2"
equation "d326 = d325"
equation "d328 = d325"
equation "d330 = d325"
equation "d331 = d325"
equation "d332 = d325"
equation "d333 = d325"
equation "d341 = d340"
equation "d342 = d340"
equation "d343 = d340"
equation "d344 = d340"
equation "d345 = d340"
equation "d346 = d340"
equation "d347 = d340"
equation "d371 = d35"
equation "d372 = d28"
equation "d373 = d31"
equation "d398 = d142"
equation "d400 = d393"
equation "d403 = d145"
equation "d405 = d403"
equation "d407 = d403"
equation "d408 = d395"
named bodies: "Arduino_Spot_Welder_V4_Case_Bottom", "Arduino_Spot_Welder_V4_Case_Top", "Fan_30mm"
